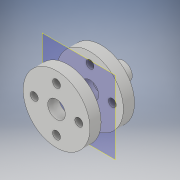
# Autodesk Inventor part: Part1
Saved by Autodesk Inventor 2019 (Build 230136000, 136)
## iProperties
Created: 2019-02-05
Part Number: Part1
Material: Generic
Document SubType Name: Modeling
Designer: UMDIEEE
Density: 1 g/cm^3
Appearance: Default
Author: UMDIEEE
Autodesk Inventor part; units mm, degrees
ref_plane "YZ Plane" through (0, 0, 0) normal (1, 0, 0) x (0, 1, 0)
ref_plane "XZ Plane" through (0, 0, 0) normal (0, 1, 0) x (-1, 0, 0)
ref_plane "XY Plane" through (0, 0, 0) normal (0, 0, 1) x (1, 0, 0)
sketch "Sketch1" plane through (0, 0, 0) normal (0, 0, 1) x (1, 0, 0)
  circle A0 centre (0, 0) radius 9.5
  circle A1 centre (0, 0) radius 2.5
  circle A2 centre (-6.35, 0) radius 1.1303
  circle A3 centre (0, 6.35) radius 1.1303
  circle A4 centre (6.35, 0) radius 1.1303
  circle A5 centre (0, -6.35) radius 1.1303
  dimension "d0" = 19
  dimension "d1" = 5
  dimension "d2" = 6.35
  dimension "d3" = 2.2606
  dimension "d4" = 6.35
  dimension "d5" = 6.35
  dimension "d6" = 6.35
  dimension "d7" = 2.2606
  dimension "d8" = 2.2606
  dimension "d9" = 2.2606
  constraints: 6 centre point, 2 coincident
  measures "d0" diameter of A0
  measures "d1" diameter of A1
  measures "d2" distance of point (0, 0) A2.centre
  measures "d3" diameter of A2
  measures "d4" distance of point (0, 0) A3.centre
  measures "d5" distance of point (0, 0) A4.centre
  measures "d6" distance of point (0, 0) A5.centre
  measures "d7" diameter of A3
  measures "d8" diameter of A4
  measures "d9" diameter of A5
extrude "Extrusion1" add sketch "Sketch1" along normal blind 3.175
ref_plane "Work Plane1" through (0, 0, -3.175) normal (0, 0, -1) x (-1, 0, 0)
mirror "Mirror1" about plane through (0, 0, -3.175) normal (0, 0, -1) of "Extrusion1"
sketch "Sketch2" plane through (0, 0, -9.525) normal (0, 0, -1) x (-1, 0, 0)
  circle A0 centre (0, 0) radius 2.5
  constraints: 1 centre point, 1 coincident
extrude "Extrusion2" add sketch "Sketch2" along normal blind 6.35
body "Solid1"
